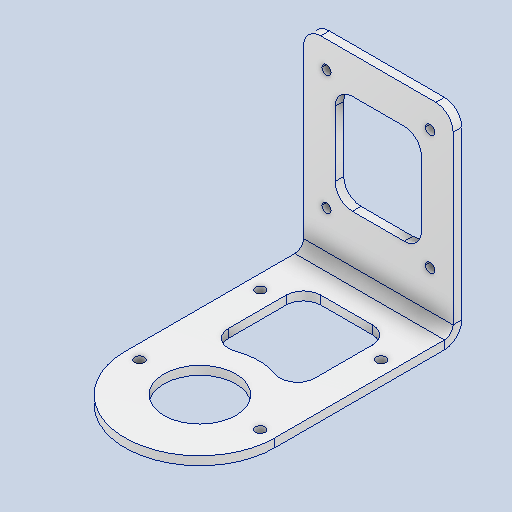
# Autodesk Inventor part: toe_back
Saved by Autodesk Inventor 2024.1 (Build 281209000, 209)
## iProperties
Created: 2024-02-12
Part Number: toe_back
Material: アルミニウム 6061
Document SubType Name: Sheet Metal
Designer: hibik
Density: 2.7 g/cm^3
Sheet Metal Rule: Default_mm
Appearance: アルミニウム - フラット
Author: hibik
Autodesk Inventor part; units mm, degrees
ref_plane "YZ Plane" through (0, 0, 0) normal (1, 0, 0) x (0, 1, 0)
ref_plane "XZ Plane" through (0, 0, 0) normal (0, 1, 0) x (-1, 0, 0)
ref_plane "XY Plane" through (0, 0, 0) normal (0, 0, 1) x (1, 0, 0)
sketch "スケッチ1" plane through (0, 0, 0) normal (0, 1, 0) x (-1, 0, 0)
  line L0 (26, 0) -> (0, 0)
  line L1 (0, 0) -> (0, -89.5474)
  line L2 (0, -89.5474) -> (26, -89.5474)
  line L3 (26, -89.5474) -> (26, 0)
  line L4 (26, 0) -> (0, 0)
  line L5 (0, 0) -> (0, 70)
  line L6 (0, 70) -> (26, 70)
  line L7 (26, 70) -> (26, 0)
  line L8 (26, 32.5) -> (0, 32.5)
  circle A0 centre (13, 32.5) radius 6.25
  circle A1 centre (13, 32.5) radius 13
  point P0 (26, 32.5)
  point P1 (0, 32.5)
  dimension "d2" = 70
  dimension "d3" = 26
  dimension "d4" = 32.5
  dimension "d5" = 12.5
  measures "d2" distance of L4.end L5.end
  measures "d3" distance of L5.end L6.end
  measures "d4" distance between parallel lines of L0 L8
  measures "d5" diameter of A0
extrude "プレート1" add sketch "スケッチ1" along normal blind 1.5 contours L0 L5 A1 L7 | A1 L8 A0 | L8 A0 A1
sketch "スケッチ2" plane through (-26, 0, 1.5) normal (0, 0, -1) x (-1, 0, 0)
  line L0 (-26, 0) -> (0, 0)
  line L1 (0, 0) -> (0, 35)
  line L2 (0, 35) -> (-26, 35)
  line L3 (-26, 35) -> (-26, 0)
  constraints: 6 end point, 1 horizontal, 1 perpendicular, 1 vertical
edge flange "フランジ1" height 35 angle 90 thickness 1.5 bend radius 1.5 thickness toward (0, 0, -1) relief straight relief width 1.5 relief depth 0.75 edges at (-13, 1.5, 0) wall of the first edge with corners at (0, 0, 1.5) (-26, 0, 1.5) (-26, 35, 1.5) (0, 35, 1.5)
bend "曲げ1"
corner "コーナー1"
sketch "スケッチ3" plane through (0, 1.5, 0) normal (0, 1, 0) x (1, 0, 0)
  circle A0 centre (-23.5, -32.5) radius 0.85 projected
  circle A1 centre (-23.5, -11.5) radius 0.85 projected
  circle A2 centre (-2.5, -11.5) radius 0.85 projected
  circle A3 centre (-2.5, -32.5) radius 0.85 projected
  point P0 (0, 0)
extrude "切り取り1" cut sketch "スケッチ3" against normal blind 1.5
sketch "スケッチ4" plane through (0, 35, 0) normal (0, 0, -1) x (-1, 0, 0)
  spline S0 degree 3 poles (4.8, -25.3846) (4.8, -25.2845) (4.78, -25.178) (4.6999, -24.983) (4.6397, -24.8944) (4.4988, -24.7507) (4.4073, -24.6876) (4.208, -24.6046) (4.1004, -24.5846) (3.8988, -24.5846) (3.7907, -24.6049) (3.5913, -24.6885) (3.4999, -24.7517) (3.3597, -24.8953) (3.2999, -24.9835) (3.22, -25.178) (3.2, -25.2844) (3.2, -25.4848) (3.22, -25.5912) (3.2999, -25.7858) (3.3597, -25.8739) (3.4999, -26.0176) (3.5913, -26.0808) (3.7907, -26.1643) (3.8988, -26.1846) (4.1004, -26.1846) (4.208, -26.1646) (4.4073, -26.0816) (4.4988, -26.0186) (4.6397, -25.8748) (4.6999, -25.7862) (4.78, -25.5912) (4.8, -25.4847) (4.8, -25.3846) knots 0 0 0 0 0.060514 0.060514 0.121029 0.121029 0.185215 0.185215 0.249402 0.249402 0.314126 0.314126 0.37885 0.37885 0.439425 0.439425 0.5 0.5 0.560575 0.560575 0.62115 0.62115 0.685874 0.685874 0.750598 0.750598 0.814785 0.814785 0.878971 0.878971 0.939486 0.939486 1 1 1 1
  spline S1 degree 3 poles (4.8, -4.6154) (4.8, -4.5153) (4.78, -4.4088) (4.6999, -4.2138) (4.6397, -4.1252) (4.4988, -3.9814) (4.4073, -3.9184) (4.208, -3.8354) (4.1004, -3.8154) (3.8988, -3.8154) (3.7907, -3.8357) (3.5913, -3.9192) (3.4999, -3.9824) (3.3597, -4.1261) (3.2999, -4.2142) (3.22, -4.4088) (3.2, -4.5152) (3.2, -4.7156) (3.22, -4.822) (3.2999, -5.0165) (3.3597, -5.1047) (3.4999, -5.2483) (3.5913, -5.3115) (3.7907, -5.3951) (3.8988, -5.4154) (4.1004, -5.4154) (4.208, -5.3954) (4.4073, -5.3124) (4.4988, -5.2493) (4.6397, -5.1056) (4.6999, -5.017) (4.78, -4.822) (4.8, -4.7155) (4.8, -4.6154) knots 0 0 0 0 0.060514 0.060514 0.121029 0.121029 0.185215 0.185215 0.249402 0.249402 0.314126 0.314126 0.37885 0.37885 0.439425 0.439425 0.5 0.5 0.560575 0.560575 0.62115 0.62115 0.685874 0.685874 0.750598 0.750598 0.814785 0.814785 0.878971 0.878971 0.939486 0.939486 1 1 1 1
  spline S2 degree 3 poles (22.8, -4.6154) (22.8, -4.5152) (22.78, -4.4088) (22.7001, -4.2142) (22.6403, -4.1261) (22.5001, -3.9824) (22.4087, -3.9192) (22.2093, -3.8357) (22.1012, -3.8154) (21.8996, -3.8154) (21.792, -3.8354) (21.5927, -3.9184) (21.5012, -3.9814) (21.3603, -4.1252) (21.3001, -4.2138) (21.22, -4.4088) (21.2, -4.5153) (21.2, -4.7155) (21.22, -4.822) (21.3001, -5.017) (21.3603, -5.1056) (21.5012, -5.2493) (21.5927, -5.3124) (21.792, -5.3954) (21.8996, -5.4154) (22.1012, -5.4154) (22.2093, -5.3951) (22.4087, -5.3115) (22.5001, -5.2483) (22.6403, -5.1047) (22.7001, -5.0165) (22.78, -4.822) (22.8, -4.7156) (22.8, -4.6154) knots 0 0 0 0 0.060575 0.060575 0.12115 0.12115 0.185874 0.185874 0.250598 0.250598 0.314785 0.314785 0.378971 0.378971 0.439486 0.439486 0.5 0.5 0.560514 0.560514 0.621029 0.621029 0.685215 0.685215 0.749402 0.749402 0.814126 0.814126 0.87885 0.87885 0.939425 0.939425 1 1 1 1
  spline S3 degree 3 poles (22.8, -25.3846) (22.8, -25.2844) (22.78, -25.178) (22.7001, -24.9835) (22.6403, -24.8953) (22.5001, -24.7517) (22.4087, -24.6885) (22.2093, -24.6049) (22.1012, -24.5846) (21.8996, -24.5846) (21.792, -24.6046) (21.5927, -24.6876) (21.5012, -24.7507) (21.3603, -24.8944) (21.3001, -24.983) (21.22, -25.178) (21.2, -25.2845) (21.2, -25.4847) (21.22, -25.5912) (21.3001, -25.7862) (21.3603, -25.8748) (21.5012, -26.0186) (21.5927, -26.0816) (21.792, -26.1646) (21.8996, -26.1846) (22.1012, -26.1846) (22.2093, -26.1643) (22.4087, -26.0808) (22.5001, -26.0176) (22.6403, -25.8739) (22.7001, -25.7858) (22.78, -25.5912) (22.8, -25.4848) (22.8, -25.3846) knots 0 0 0 0 0.060575 0.060575 0.12115 0.12115 0.185874 0.185874 0.250598 0.250598 0.314785 0.314785 0.378971 0.378971 0.439486 0.439486 0.5 0.5 0.560514 0.560514 0.621029 0.621029 0.685215 0.685215 0.749402 0.749402 0.814126 0.814126 0.87885 0.87885 0.939425 0.939425 1 1 1 1
  point P0 (0, -35)
  point P1 (4.8, -25.3846)
  point P2 (4.8, -4.6154)
  point P3 (22.8, -4.6154)
  point P4 (22.8, -25.3846)
extrude "切り取り2" cut sketch "スケッチ4" against normal blind 1.5
sketch "スケッチ5" plane through (0, 1.5, 0) normal (0, 1, 0) x (1, 0, 0)
  line L0 (-20.5, -10) -> (-20.5, -20.0376) projected
  arc A0 (-20.5, -20.0376) -> (-16.4811, -22.8592) centre (-17.5, -20.0376) ccw projected
  arc A1 (-9.5189, -22.8592) -> (-16.4811, -22.8592) centre (-13, -32.5) ccw projected
  arc A2 (-9.5189, -22.8592) -> (-5.5, -20.0376) centre (-8.5, -20.0376) ccw projected
  line L1 (-5.5, -20.0376) -> (-5.5, -10) projected
  arc A3 (-5.5, -10) -> (-8.5, -7) centre (-8.5, -10) ccw projected
  line L2 (-8.5, -7) -> (-17.5, -7) projected
  arc A4 (-17.5, -7) -> (-20.5, -10) centre (-17.5, -10) ccw projected
  line L3 (-26, -3) -> (0, -3) projected
  line L4 (0, -32.5) -> (0, -3) projected
  arc A5 (-26, -32.5) -> (0, -32.5) centre (-13, -32.5) ccw projected
  line L5 (-26, -3) -> (-26, -32.5) projected
  circle A6 centre (-13, -32.5) radius 6.25 projected
  circle A7 centre (-23.5, -32.5) radius 0.85 projected
  circle A8 centre (-2.5, -11.5) radius 0.85 projected
  circle A9 centre (-2.5, -32.5) radius 0.85 projected
  circle A10 centre (-23.5, -11.5) radius 0.85 projected
  point P0 (0, 0)
extrude "切り取り3" cut sketch "スケッチ5" against normal blind 1.5 contours A4 L2 A3 L1 A2 A1 A0 L0
sketch "スケッチ6" plane through (0, 35, 0) normal (0, 0, -1) x (-1, 0, 0)
  line L0 (26, 0) -> (26, -32) projected
  line L1 (0, 0) -> (26, 0) projected
  line L2 (0, -32) -> (0, 0) projected
  circle A0 centre (22, -25.3846) radius 0.8 projected
  circle A1 centre (4, -25.3846) radius 0.8 projected
  circle A2 centre (4, -4.6154) radius 0.8 projected
  circle A3 centre (22, -4.6154) radius 0.8 projected
  line L3 (22, -25.3846) -> (4, -4.6154)
  line L4 (4, -25.3846) -> (22, -4.6154)
  line L5 (17.5, -23.6538) -> (8.5, -23.6538)
  line L6 (5.5, -20.6538) -> (5.5, -9.3462)
  line L7 (8.5, -6.3462) -> (17.5, -6.3462)
  line L8 (20.5, -9.3462) -> (20.5, -20.6538)
  arc A4 (26, -3) -> (23, 0) centre (23, -3) ccw
  line L9 (0, 0) -> (26, 0) projected
  arc A5 (3, 0) -> (0, -3) centre (3, -3) ccw
  arc A6 (17.5, -23.6538) -> (20.5, -20.6538) centre (17.5, -20.6538) ccw
  arc A7 (5.5, -20.6538) -> (8.5, -23.6538) centre (8.5, -20.6538) ccw
  arc A8 (8.5, -6.3462) -> (5.5, -9.3462) centre (8.5, -9.3462) ccw
  arc A9 (20.5, -9.3462) -> (17.5, -6.3462) centre (17.5, -9.3462) ccw
  point P0 (0, -35)
  point P1 (20.5, -23.6538)
  point P2 (5.5, -6.3462)
  point P3 (5.5, -23.6538)
  dimension "d29" = 1.5
  dimension "d30" = 3
  dimension "d31" = 3
  dimension "d32" = 3
  constraints: 14 point on line, 12 end point, 12 point on circle, 12 tangent, 6 centre point, 3 equal radius, 2 parallel, 1 horizontal, 1 perpendicular
  measures "d29" distance from line of L3.start L8
  measures "d30" radius of A4
  measures "d31" radius of A5
  measures "d32" radius of A6
extrude "切り取り4" cut sketch "スケッチ6" against normal blind 1.5 contours L0 A4 L1 | L1 A5 L2 | A6 L5 A7 L4 L3 | L3 L4 A9 L8 A6 | L4 A7 L6 A8 L3 | L3 A8 L7 A9 L4
equation "\"d23\" = Thickness"
equation "\"d25\" = Thickness"
equation "\"d27\" = Thickness"
equation "\"d33\" = Thickness"
equation "\"d12\" = Thickness"
equation "\"d13\" = BendReliefWidth"
equation "\"d14\" = BendReliefDepth"
equation "\"d15\" = MinimumRemnant"
equation "\"d16\" = TransitionRadius"
equation "\"d19\" = BendRadius"
equation "\"d20\" = CornerReliefSize"
equation "\"d21\" = GapSize"
equation "\"d22\" = JacobiRadiusSize"
equation "\"BendRadius\" = Thickness"
equation "\"BendReliefWidth\" = Thickness"
equation "\"BendReliefDepth\" = 0.5 * Thickness"
equation "\"CornerReliefSize\" = 4 * Thickness"
equation "\"MinimumRemnant\" = 2 * Thickness"
equation "\"TransitionRadius\" = BendRadius"
equation "\"JacobiRadiusSize\" = BendRadius"
equation "\"GapSize\" = Thickness"
equation "\"Thickness\" = 1.5"
